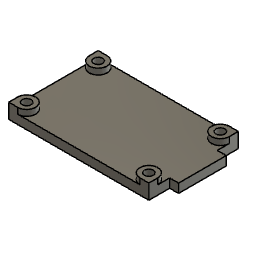
usb2uart_lid (Autodesk Fusion 360 design; units mm, degrees)
Autodesk Fusion 360 part; units mm, degrees
sketch "Sketch1" plane through (0, 0, 0) normal (0, 1, 0) x (1, 0, 0)
  line L0 (0, 0) -> (47, 0)
  line L1 (47, 0) -> (47, -30)
  line L2 (47, -30) -> (0, -30)
  line L3 (0, -30) -> (0, 0)
  line L4 (47, -7.029) -> (50, -7.029)
  line L5 (50, -7.029) -> (50, -23.029)
  line L6 (50, -23.029) -> (47, -23.029)
  line L7 (47, -23.029) -> (47, -7.029)
  dimension "d1" = 47
  dimension "d2" = 30
  dimension "d3" = 16
  constraint horizontal L0
  constraint vertical L1
  constraint horizontal L2
  constraint vertical L3
  constraint coincident L0.start L3.end
  constraint horizontal L4
  constraint vertical L5
  constraint horizontal L6
  constraint vertical L7
  constraint coincident L1 L4.start
  measures "d1" distance of L0.start L0.end
  measures "d2" distance of L0.start L2.end
  measures "d3" distance of L4.start L6.end
extrude "Extrude1" add sketch "Sketch1" along normal blind 3
sketch "Sketch2" plane through (0, 3, 0) normal (0, 1, 0) x (-1, 0, 0)
  line L0 (-50, 23.029) -> (-50, 7.029)
  line L1 (-50, 7.029) -> (-47, 7.029)
  line L2 (-47, 7.029) -> (-47, 0)
  line L3 (-47, 0) -> (0, 0)
  line L4 (0, 0) -> (0, 30)
  line L5 (0, 30) -> (-47, 30)
  line L6 (-47, 30) -> (-47, 23.029)
  line L7 (-47, 23.029) -> (-50, 23.029)
  line L8 (-50, 23.029) -> (-47, 23.029)
  line L9 (-47, 23.029) -> (-47, 7.029)
  line L10 (-47, 7.029) -> (-50, 7.029)
  line L11 (-50, 7.029) -> (-50, 23.029)
  line L12 (-47, 30) -> (0, 30)
  line L13 (0, 30) -> (0, 0)
  line L14 (0, 0) -> (-47, 0)
  line L15 (-47, 0) -> (-47, 30)
  circle A0 centre (-44, 27) radius 3
  circle A1 centre (-3, 27) radius 3
  circle A2 centre (-44, 3) radius 3
  circle A3 centre (-3, 3) radius 3
  circle A4 centre (-3, 3) radius 1.5
  circle A5 centre (-44, 3) radius 1.5
  circle A6 centre (-44, 27) radius 1.5
  circle A7 centre (-3, 27) radius 1.5
  dimension "d6" = 6
  dimension "d7" = 3
  dimension "d8" = 3
  dimension "d9" = 3
  constraint horizontal L8
  constraint vertical L9
  constraint horizontal L10
  constraint vertical L11
  constraint coincident L1.end L2.start
  constraint coincident L0.start L7.end
  constraint horizontal L12
  constraint vertical L13
  constraint horizontal L14
  constraint vertical L15
  constraint coincident L3.end L4.start
  constraint coincident L5.end L6.start
  constraint tangent L6 A0
  constraint tangent L3 A2
  constraint tangent L14 A3
  constraint concentric A3 A4
  constraint concentric A2 A5
  constraint concentric A0 A6
  constraint concentric A1 A7
  measures "d6" diameter of A1
  measures "d7" diameter of A4
  measures "d8" diameter of A5
  measures "d9" diameter of A7
extrude "Extrude2" add sketch "Sketch2" along normal blind 2 contours L5 L6 L12 L15 A0 | A0 | L2 L3 L14 L15 A2 | A2 | L4 L5 L12 L13 A1 | A1 | L3 L4 L13 L14 A3 | A3
sketch "Sketch3" plane through (0, 0, 0) normal (0, -1, 0) x (1, 0, 0)
  line L0 (50, 7.029) -> (50, 23.029)
  line L1 (50, 23.029) -> (47, 23.029)
  line L2 (47, 23.029) -> (47, 30)
  line L3 (47, 30) -> (0, 30)
  line L4 (0, 30) -> (0, 0)
  line L5 (0, 0) -> (47, 0)
  line L6 (47, 0) -> (47, 7.029)
  line L7 (47, 7.029) -> (50, 7.029)
  circle A0 centre (3, 27) radius 3
  circle A1 centre (3, 27) radius 1.5
  circle A2 centre (44, 27) radius 3
  circle A3 centre (44, 27) radius 1.5
  circle A4 centre (3, 3) radius 3
  circle A5 centre (3, 3) radius 1.5
  circle A6 centre (44, 3) radius 3
  circle A7 centre (44, 3) radius 1.5
  dimension "d12" = 6
  dimension "d13" = 3
  dimension "d14" = 6
  dimension "d15" = 3
  constraint tangent L4 A0
  constraint concentric A0 A1
  constraint concentric A2 A3
  constraint tangent L5 A4
  constraint concentric A4 A5
  constraint tangent L6 A6
  constraint concentric A6 A7
  measures "d12" diameter of A0
  measures "d13" diameter of A1
  measures "d14" diameter of A2
  measures "d15" diameter of A5
extrude "Extrude3" cut sketch "Sketch3" against normal blind 6 contours A1 | A3 | A5 | A7
chamfer "Chamfer1" distance 1 angle 45 1 edges at (1.6015, 0, 3.5424)
chamfer "Chamfer2" distance 1 angle 45 1 edges at (42.6015, 0, 3.5424)
chamfer "Chamfer3" distance 1 angle 45 1 edges at (1.6015, 0, 27.5424)
chamfer "Chamfer4" distance 1 angle 45 1 edges at (42.6015, 0, 27.5424)
